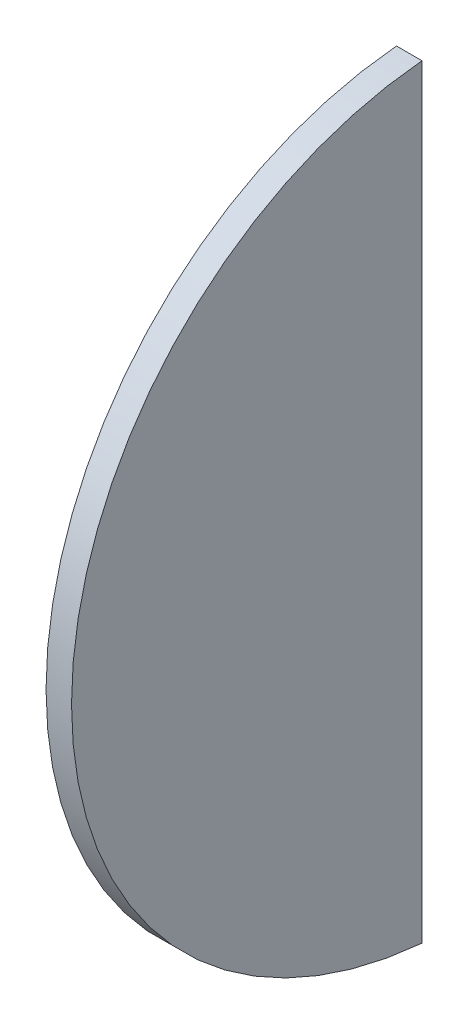
# Autodesk Inventor part: Lid2
Saved by Autodesk Inventor 2026 (Build 300175050, 175E)
## iProperties
Created: 2025-08-01
Part Number: Lid2
Material: Plastic, Opaque White
Document SubType Name: Modeling
Designer: Cupri
Mass: 37.7239 g
Surface Area: 177.179 cm^2
Volume: 39.626 cm^3
Density: 0.952 g/cm^3
Appearance: Smooth - White
Author: Cupri
Autodesk Inventor part; units mm, degrees
ref_plane "YZ Plane" through (0, 0, 0) normal (1, 0, 0) x (0, 1, 0)
ref_plane "XZ Plane" through (0, 0, 0) normal (0, 1, 0) x (-1, 0, 0)
ref_plane "XY Plane" through (0, 0, 0) normal (0, 0, 1) x (1, 0, 0)
ref_plane "Work Plane1" through (-2.5, 0, 34.3925) normal (1, 0, 0) x (0, 1, 0)
sketch "Sketch1" plane through (-2.5, 0, 34.3925) normal (1, 0, 0) x (0, 1, 0)
  arc A0 (72.5, -34.3925) -> (-72.5, -34.3925) centre (0, -45.8883) ccw projected
  line L0 (72.5, -34.3925) -> (67.5, -34.3925) projected
  line L1 (67.5, -34.3925) -> (-67.5, -34.3925) projected
  line L2 (-72.5, -34.3925) -> (-67.5, -34.3925) projected
  line L3 (67.5, -34.3925) -> (-67.5, -34.3925) projected
  arc A1 (75, -34.3925) -> (-75, -34.3925) centre (0, -40.8883) ccw projected
  line L4 (-72.5, -34.3925) -> (-75, -34.3925) projected
  arc A2 (72.5, -34.3925) -> (-72.5, -34.3925) centre (0, -45.8883) ccw projected
  line L5 (75, -34.3925) -> (72.5, -34.3925) projected
  point P0 (0, -34.3925)
ref_plane "Work Plane2" through (2.5, -67.5, -250) normal (1, 0, 0) x (0, 1, 0)
ref_plane "Work Plane3" through (-2.5, -72.3, -250) normal (-1, 0, 0) x (0, 0, 1)
extrude "Extrusion1" add sketch "Sketch1" against normal up to surface (5 mm away) from surface at 5
body "Solid1"
